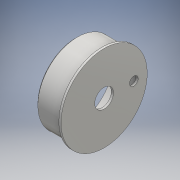
# Autodesk Inventor part: aftPlug
Saved by Autodesk Inventor 2016 (Build 200138000, 138)
## iProperties
Created: 2015-11-15
Part Number: aftPlug
Material: PVC-Piping
Document SubType Name: Modeling
Designer: Artur
Density: 1.4 g/cm^3
Appearance: Smooth - White
Mass: 85.2175 g
Surface Area: 461.19 cm^2
Volume: 60.8697 cm^3
Author: Artur
Autodesk Inventor part; units mm, degrees
ref_plane "YZ Plane" through (0, 0, 0) normal (1, 0, 0) x (0, 1, 0)
ref_plane "XZ Plane" through (0, 0, 0) normal (0, 1, 0) x (-1, 0, 0)
ref_plane "XY Plane" through (0, 0, 0) normal (0, 0, 1) x (1, 0, 0)
sketch "Sketch1" plane through (0, 0, 0) normal (0, 1, 0) x (-1, 0, 0)
  line L0 (0, 0) -> (0, -59.5)
  line L1 (0, -59.5) -> (3, -59.5)
  line L2 (3, -59.5) -> (3, -54.5)
  line L3 (3, -54.5) -> (39, -54.5)
  line L4 (39, -54.5) -> (39, -52)
  line L5 (39, -52) -> (3, -52)
  line L6 (3, -52) -> (3, 0)
  line L7 (3, 0) -> (0, 0)
  dimension "d3" = 3
  dimension "d4" = 5
  dimension "d5" = 36
  dimension "d6" = 2.5
  dimension "d14" = 52
  constraints: 16 end point, 5 perpendicular, 2 point on line, 1 horizontal, 1 vertical
  measures "d3" distance of L0.end L1.end
  measures "d4" distance of L1.end L2.end
  measures "d5" distance of L2.end L3.end
  measures "d6" distance of L3.end L4.end
  measures "d14" distance from line of L0.start L5
revolve "Revolution1" add sketch "Sketch1" angle 360 about axis through (-3, 0, 0) along (1, 0, 0)
chamfer "Chamfer1" distance 2 angle 45 1 edges at (-39, 0, 54.5)
sketch "Sketch3" plane through (0, 0, 0) normal (1, 0, 0) x (0, 0, -1)
  circle A0 centre (0, 0) radius 13
  circle A1 centre (0, 0) radius 52 construction
  line L0 (0, 0) -> (0, 103.7887) construction
  circle A2 centre (0, 41) radius 6
  point P0 (0, 52)
  dimension "d15" = 26
  dimension "d16" = 12
  dimension "d17" = 11
  constraints: 2 centre point, 2 end point, 2 point on line, 1 coincident, 1 vertical, 1 vertical alignment, 1 other
  measures "d15" diameter of A0
  measures "d16" diameter of A2
  measures "d17" distance of A2.centre point (0, 52)
extrude "holes" cut sketch "Sketch3" against normal blind 10
body "Solid1"
